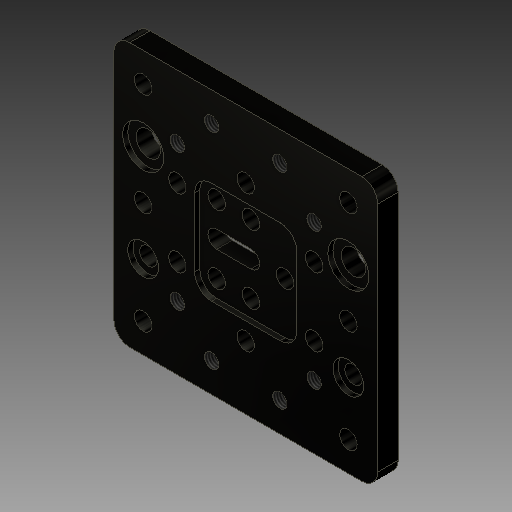
# Autodesk Inventor part: C-Beam Gantry Plate
Saved by Autodesk Inventor 2019 (Build 230136000, 136)
## iProperties
Created: 2020-11-06
Part Number: C-Beam Gantry Plate
Material: Aluminum 6061
Document SubType Name: Modeling
Designer: asus
Density: 2.7 g/cm^3
Appearance: Gunmetal
Author: asus
Autodesk Inventor part; units mm, degrees
ref_plane "YZ Plane" through (0, 0, 0) normal (1, 0, 0) x (0, 1, 0)
ref_plane "XZ Plane" through (0, 0, 0) normal (0, 1, 0) x (-1, 0, 0)
ref_plane "XY Plane" through (0, 0, 0) normal (0, 0, 1) x (1, 0, 0)
sketch "Sketch1" plane through (0, 0, 0) normal (0, 0, 1) x (1, 0, 0)
  line L0 (-33.935, -38.575) -> (33.935, -38.575)
  line L1 (38.575, -33.935) -> (38.575, 33.935)
  line L2 (33.935, 38.575) -> (-33.935, 38.575)
  line L3 (-38.575, 33.935) -> (-38.575, -33.935)
  arc A0 (-33.935, 38.575) -> (-38.575, 33.935) centre (-33.935, 33.935) ccw
  arc A1 (38.575, 33.935) -> (33.935, 38.575) centre (33.935, 33.935) ccw
  arc A2 (-38.575, -33.935) -> (-33.935, -38.575) centre (-33.935, -33.935) ccw
  arc A3 (33.935, -38.575) -> (38.575, -33.935) centre (33.935, -33.935) ccw
  circle A4 centre (-30, 30) radius 2.55
  circle A5 centre (-10, 30) radius 2.1
  circle A6 centre (9.97, 30) radius 2.1
  circle A7 centre (30, 30) radius 2.55
  circle A8 centre (-30, 14.25) radius 3.6
  circle A9 centre (-20, 20) radius 2.1
  circle A10 centre (20, 20) radius 2.1
  circle A11 centre (0, 20) radius 2.55
  circle A12 centre (20, 10) radius 2.55
  circle A13 centre (-20, 10) radius 2.55
  circle A14 centre (-10, 10) radius 2.55
  circle A15 centre (0, 10) radius 2.55
  circle A16 centre (30, 14.25) radius 3.6
  circle A17 centre (-30, 0) radius 2.55
  circle A18 centre (-30, -14.25) radius 2.55
  circle A19 centre (-30, -30) radius 2.55
  circle A20 centre (9.97, 0) radius 2.55
  circle A21 centre (30, 0) radius 2.55
  line L4 (0, 0) -> (-10, 0) construction
  line L5 (0, 2.55) -> (-10, 2.55)
  line L6 (-10, -2.55) -> (0, -2.55)
  arc A22 (0, -2.55) -> (0, 2.55) centre (0, 0) ccw
  arc A23 (-10, 2.55) -> (-10, -2.55) centre (-10, 0) ccw
  circle A24 centre (-10, -30) radius 2.1
  circle A25 centre (9.97, -30) radius 2.1
  circle A26 centre (30, -30) radius 2.55
  circle A27 centre (-20, -20) radius 2.1
  circle A28 centre (20, -20) radius 2.1
  circle A29 centre (0, -20) radius 2.55
  circle A30 centre (20, -10) radius 2.55
  circle A31 centre (-20, -10) radius 2.55
  circle A32 centre (-10, -10) radius 2.55
  circle A33 centre (0, -10) radius 2.55
  circle A34 centre (30, -14.25) radius 2.55
  point P0 (0, 0)
  point P1 (38.575, 38.575)
  point P2 (38.575, -38.575)
  point P3 (-38.575, 38.575)
  point P4 (38.575, 0)
  point P5 (0, 38.575)
  point P6 (-5, 0)
  dimension "d0" = 77.15
  dimension "d1" = 77.15
  dimension "d2" = 4.64
  dimension "d3" = 5.1
  dimension "d4" = 4.2
  dimension "d5" = 8.575
  dimension "d6" = 18.575
  dimension "d7" = 8.575
  dimension "d8" = 7.2
  dimension "d9" = 24.325
  dimension "d10" = 38.575
  dimension "d11" = 52.825
  dimension "d12" = 68.575
  dimension "d13" = 28.575
  dimension "d14" = 18.575
  dimension "d15" = 38.575
  dimension "d16" = 48.545
  dimension "d17" = 58.575
  dimension "d18" = 68.575
  dimension "d19" = 28.575
  dimension "d20" = 10
  dimension "d21" = 5.1
  dimension "d22" = 5.1
  constraints: 35 centre point, 18 equal radius, 16 end point, 14 horizontal alignment, 14 vertical alignment, 12 point on circle, 12 tangent, 10 symmetric about line, 6 point on line, 3 midpoint, 3 parallel, 2 horizontal, 1 perpendicular, 10 other
  measures "d0" distance of point (-38.575, 38.575) point (38.575, 38.575)
  measures "d1" distance of point (38.575, 38.575) point (38.575, -38.575)
  measures "d2" radius of A0
  measures "d3" diameter of A7
  measures "d4" diameter of A6
  measures "d5" distance from line of L2 A5.centre
  measures "d6" distance from line of L2 A9.centre
  measures "d7" distance from line of L3 A4.centre
  measures "d8" diameter of A8
  measures "d9" distance from line of L2 A8.centre
  measures "d10" distance from line of L2 A17.centre
  measures "d11" distance from line of L2 A18.centre
  measures "d12" distance from line of L2 A19.centre
  measures "d13" distance from line of L3 A5.centre
  measures "d14" distance from line of L3 A9.centre
  measures "d15" distance from line of L3 A11.centre
  measures "d16" distance from line of L3 A6.centre
  measures "d17" distance from line of L3 A10.centre
  measures "d18" distance from line of L3 A7.centre
  measures "d19" distance from line of L2 A13.centre
  measures "d20" distance of L4.start L4.end
  measures "d21" diameter of A23
  measures "d22" diameter of A34
extrude "Extrusion1" add sketch "Sketch1" along normal blind 6
sketch "Sketch2" plane through (0, 0, 6) normal (0, 0, 1) x (1, 0, 0)
  circle A0 centre (-30, 14.25) radius 3.6 projected
  circle A1 centre (30, 14.25) radius 3.6 projected
  circle A2 centre (-30, -14.25) radius 2.55 projected
  circle A3 centre (30, -14.25) radius 2.55 projected
  circle A4 centre (-30, 14.25) radius 6
  circle A5 centre (-30, -14.25) radius 4.5
  circle A6 centre (30, -14.25) radius 4.5
  circle A7 centre (30, 14.25) radius 6
  line L0 (-10.025, 14.945) -> (10.035, 14.945)
  line L1 (14.955, 10.025) -> (14.955, -10.035)
  line L2 (10.035, -14.955) -> (-10.025, -14.955)
  line L3 (-14.945, -10.035) -> (-14.945, 10.025)
  line L4 (-38.575, 33.935) -> (-38.575, -33.935) projected
  line L5 (33.935, 38.575) -> (-33.935, 38.575) projected
  arc A8 (-14.945, -10.035) -> (-10.025, -14.955) centre (-10.025, -10.035) ccw
  arc A9 (10.035, -14.955) -> (14.955, -10.035) centre (10.035, -10.035) ccw
  arc A10 (14.955, 10.025) -> (10.035, 14.945) centre (10.035, 10.025) ccw
  arc A11 (-10.025, 14.945) -> (-14.945, 10.025) centre (-10.025, 10.025) ccw
  point P0 (0, 0)
  dimension "d25" = 12
  dimension "d26" = 9
  dimension "d27" = 23.63
  dimension "d28" = 53.53
  dimension "d29" = 23.63
  dimension "d30" = 53.53
  dimension "d31" = 4.92
  constraints: 8 centre point, 8 end point, 8 point on circle, 8 tangent, 5 equal radius, 4 coincident, 2 parallel, 1 horizontal, 1 perpendicular
  measures "d25" diameter of A4
  measures "d26" diameter of A5
  measures "d27" distance between parallel lines of L4 L3
  measures "d28" distance between parallel lines of L4 L1
  measures "d29" distance between parallel lines of L5 L0
  measures "d30" distance between parallel lines of L5 L2
  measures "d31" radius of A8
extrude "Extrusion2" cut sketch "Sketch2" against normal blind 1.5
thread "Thread1" size "M5x0.8" class "6H" standard "ANSI Metric M Profile" full length
thread "Thread2" size "M5x0.8" class "6H" standard "ANSI Metric M Profile" full length
thread "Thread3" size "M5x0.8" class "6H" standard "ANSI Metric M Profile" full length
thread "Thread4" size "M5x0.8" class "6H" standard "ANSI Metric M Profile" full length
thread "Thread5" size "M5x0.8" class "6H" standard "ANSI Metric M Profile" full length
thread "Thread6" size "M5x0.8" class "6H" standard "ANSI Metric M Profile" full length
thread "Thread7" size "M5x0.8" class "6H" standard "ANSI Metric M Profile" full length
thread "Thread8" size "M5x0.8" class "6H" standard "ANSI Metric M Profile" full length
body "Solid1"
